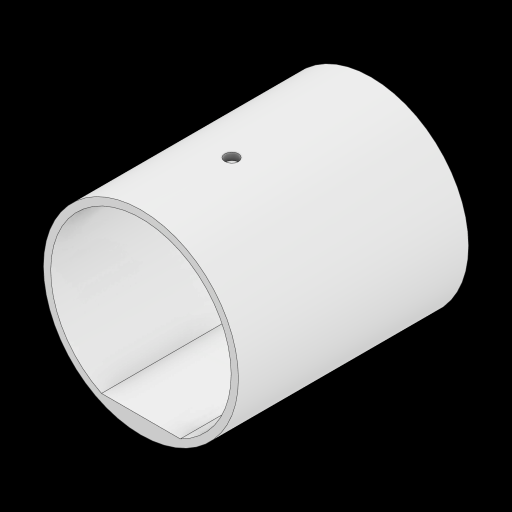
# Autodesk Inventor part: FrontTubeV1
Saved by Autodesk Inventor 2024 (Build 280153000, 153)
## iProperties
Created: 2026-04-10
Part Number: FrontTubeV1
Material: PVC-Piping
Document SubType Name: Modeling
Designer: Tanner
Density: 1.4 g/cm^3
Appearance: Smooth - White
Author: Tanner
## iProperties of the stored document FrontTubeV1_3DPrint.ipt
Created: 2026-04-13
Part Number: FrontTubeV1_3DPrint
Material: Generic
Document SubType Name: Modeling
Designer: Tanner
Density: 1 g/cm^3
Appearance: Default
Author: Tanner
Autodesk Inventor part; units mm, degrees
ref_plane "YZ Plane" through (0, 0, 0) normal (1, 0, 0) x (0, 1, 0)
ref_plane "XZ Plane" through (0, 0, 0) normal (0, 1, 0) x (-1, 0, 0)
ref_plane "XY Plane" through (0, 0, 0) normal (0, 0, 1) x (1, 0, 0)
sketch "Sketch1" plane through (0, 0, 0) normal (0, 0, 1) x (1, 0, 0)
  circle A0 centre (0, 0) radius 99.6
  circle A1 centre (0, 0) radius 107.6
  dimension "d0" = 199.2
  dimension "d1" = 8
  constraints: 2 centre point, 2 coincident
  measures "d0" diameter of A0
  measures "d1" radial gap between concentric circles of A1 A0
extrude "Extrusion1" add sketch "Sketch1" along normal blind 254
sketch "Sketch3" plane through (0, 0, 0) normal (0, 0, -1) x (-1, 0, 0)
  circle A0 centre (0, 0) radius 107.6 construction
  circle A1 centre (0, 0) radius 99.6 construction
  arc A2 (-43.4971, -89.6) -> (43.4971, -89.6) centre (0, 0) ccw
  line L0 (0, -99.6) -> (0, -89.6) construction
  line L1 (43.4971, -89.6) -> (-43.4971, -89.6)
  dimension "d11" = 10
  constraints: 5 point on circle, 4 end point, 2 concentric, 2 horizontal alignment, 1 centre point, 1 horizontal, 1 vertical
  measures "d11" distance of L0.start L0.end
extrude "Extrusion3" add sketch "Sketch3" against normal up to surface (254 mm away)
sketch "Sketch4" plane through (0, 0, 0) normal (0, 1, 0) x (-1, 0, 0)
  circle A0 centre (0, 154) radius 7.5
  line L0 (107.6, 254) -> (-107.6, 254) construction
  line L1 (107.6, 0) -> (-107.6, 0) construction
  point P0 (0, 0)
  point P1 (0, 0)
  dimension "d14" = 15
  dimension "d15" = 100
  constraints: 1 centre point, 1 midpoint, 1 vertical alignment
  measures "d14" diameter of A0
  measures "d15" distance from line of L0 A0.centre
extrude "Extrusion4" cut sketch "Sketch4" along normal up to surface
body "Solid1"
